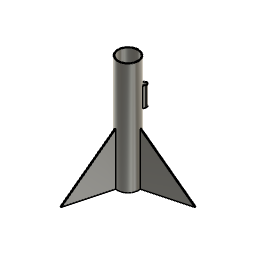
light c11 v1 (Autodesk Fusion 360 design; units mm, degrees)
Autodesk Fusion 360 part; units mm, degrees
sketch "Sketch1" plane through (0, 0, 0) normal (0, 0, 1) x (1, 0, 0)
  circle A0 centre (0, 0) radius 12.5
  circle A1 centre (0, 0) radius 14.5
  line L0 (-110, 110) -> (110, 110)
  line L1 (110, 110) -> (110, -110)
  line L2 (110, -110) -> (-110, -110)
  line L3 (-110, -110) -> (-110, 110)
  line L4 (-110, 110) -> (110, -110) construction
  line L5 (110, 110) -> (-110, -110) construction
  line L6 (-60, 60) -> (-60.3536, 59.6464)
  line L7 (-60.7071, 59.2929) -> (-59.6464, 60.3536)
  line L8 (-58.9393, 60.3536) -> (0.7071, 0.7071)
  line L9 (-60.3536, 58.9393) -> (-0.7071, -0.7071)
  arc A2 (-58.9393, 60.3536) -> (-59.6464, 60.3536) centre (-59.2929, 60) ccw
  arc A3 (-60.3536, 59.6464) -> (-60.3536, 58.9393) centre (-60, 59.2929) ccw
  line L10 (-20.9956, -82.2203) -> (-22.4445, -81.8321)
  arc A4 (-21.4786, -82.0909) -> (-20.8662, -81.7374) centre (-21.3492, -81.608) ccw
  line L11 (-20.8662, -81.7374) -> (0.9659, -0.2588)
  arc A5 (-22.798, -81.2197) -> (-22.4445, -81.8321) centre (-22.3151, -81.3492) ccw
  line L12 (-22.798, -81.2197) -> (-0.9659, 0.2588)
  line L13 (81.7027, 22.9275) -> (82.0909, 21.4786)
  arc A6 (81.8321, 22.4445) -> (81.2197, 22.798) centre (81.3492, 22.3151) ccw
  line L14 (81.2197, 22.798) -> (-0.2588, 0.9659)
  arc A7 (81.7374, 20.8662) -> (82.0909, 21.4786) centre (81.608, 21.3492) ccw
  line L15 (81.7374, 20.8662) -> (0.2588, -0.9659)
  point P0 (-59.2929, 60.7071)
  dimension "d1" = 25
  dimension "d2" = 29
  dimension "d3" = 220
  dimension "d4" = 220
  dimension "d5" = 1
  dimension "d6" = 2
  dimension "d7" = 180
  dimension "d8" = 0.5
  dimension "d10" = 360
  constraint coincident A0.centre A1.centre
  constraint horizontal L0
  constraint perpendicular L0 L1
  constraint parallel L0 L2
  constraint parallel L1 L3
  constraint coincident L4 A0.centre
  constraint coincident L5 A0.centre
  constraint coincident L4 L6.start
  constraint perpendicular L4 L6
  constraint perpendicular L4 L7
  constraint coincident L5 L8.end
  constraint perpendicular L5 L8
  constraint coincident L5 L9.end
  constraint coincident P0 L7
  constraint coincident P0 L8
  constraint tangent L7 A2
  constraint tangent L8 A2
  constraint coincident L7.start L6
  constraint coincident L7.start L9
  constraint tangent L6 A3
  constraint tangent L9 A3
  constraint equal A2 A3
  measures "d1" diameter of A0
  measures "d2" diameter of A1
  measures "d3" distance of L1.end L2.end
  measures "d4" distance of L0.end L1.end
  measures "d5" distance of L6.start L7.start
  measures "d6" distance of L7.start P0
  measures "d7" angle of L8 L9
  measures "d8" radius of A2
extrude "Extrude1" add sketch "Sketch1" along normal blind 70 contours A0 A1 L11 L15 | A0 A1 L14 L15 | A0 A1 L11 L12 | A0 A1 L8 L14 | A0 A1 L9 L12 | A0 A1 L8 L9 makes body 1
sketch "Sketch2" plane through (0, 0, 70) normal (0, 0, 1) x (-1, 0, 0)
  circle A0 centre (0, 0) radius 12.5
  circle A1 centre (0, 0) radius 14.5
  circle A2 centre (0, 0) radius 11
  dimension "d13" = 22
  constraint coincident A0.centre A1.centre
  measures "d13" diameter of A2
extrude "Extrude2" add sketch "Sketch2" along normal blind 2 contours A0 | A1 bodies 1
sketch "Sketch3" plane through (0, 0, 72) normal (0, 0, 1) x (-1, 0, 0)
  circle A0 centre (0, 0) radius 11
  circle A1 centre (0, 0) radius 14.5
  circle A2 centre (0, 0) radius 13.5
  circle A3 centre (0, 0) radius 15
  circle A4 centre (0, 0) radius 16
  dimension "d16" = 27
  dimension "d17" = 30
  dimension "d18" = 32
  constraint coincident A0.centre A1.centre
  constraint concentric A2 A4
  measures "d16" diameter of A2
  measures "d17" diameter of A3
  measures "d18" diameter of A4
extrude "Extrude3" add sketch "Sketch3" along normal blind 100 separate body contours A4 makes body 2
extrude "Extrude4" add sketch "Sketch3" against normal blind 72 contours A3 | A4 bodies 1 2
extrude "Extrude5" add sketch "Sketch1" along normal blind 80 contours A1 L13 A6 L14 A7 L15 | A1 L10 A4 L11 A5 L12 | A1 L6 L7 L8 L9 A2 A3 bodies 1
sketch "Sketch4" plane through (-0.9659, 0.2588, 0) normal (-0.965926, 0.258819, 0) x (-0.258819, -0.965926, 0)
  line L0 (15.9687, 80) -> (15.9687, 0)
  line L1 (15.9687, 0) -> (84.3528, 0)
  line L2 (84.3528, 0) -> (84.3528, 80)
  line L3 (84.3528, 80) -> (15.9687, 80)
  line L4 (15.9687, 80) -> (84.3528, 0)
  line L5 (15.9687, 80) -> (86.3566, 117.9716)
  line L6 (86.3566, 117.9716) -> (140, 40)
  line L7 (140, 40) -> (84.3528, 0)
  constraint coincident L0.start L3.end
  constraint coincident L1.end L2.start
extrude "Extrude6" cut sketch "Sketch4" against normal blind 50 contours L2 L3 L5 L6 L7 | L2 L3 L4 bodies 1
sketch "Sketch5" plane through (-0.7071, -0.7071, 0) normal (-0.707107, -0.707107, 0) x (0.707107, -0.707107, 0)
  line L0 (-15.9687, 0) -> (-15.9687, 80)
  line L1 (-15.9687, 80) -> (-84.3528, 80)
  line L2 (-84.3528, 80) -> (-84.3528, 0)
  line L3 (-84.3528, 0) -> (-15.9687, 0)
  line L4 (-15.9687, 80) -> (-84.3528, 0)
  line L5 (-84.3528, 0) -> (-114.2811, 30.3018)
  line L6 (-114.2811, 30.3018) -> (-99.317, 93.7517)
  line L7 (-99.317, 93.7517) -> (-15.9687, 80)
  constraint coincident L0.end L1.start
  constraint coincident L2.end L3.start
extrude "Extrude7" cut sketch "Sketch5" against normal blind 5 contours L1 L2 L4 | L1 L2 L5 L6 L7 bodies 1
sketch "Sketch6" plane through (-0.2588, 0.9659, 0) normal (-0.258819, 0.965926, 0) x (-0.965926, -0.258819, 0)
  line L0 (-15.9687, 0) -> (-15.9687, 80)
  line L1 (-15.9687, 80) -> (-84.3528, 80)
  line L2 (-84.3528, 80) -> (-84.3528, 0)
  line L3 (-84.3528, 0) -> (-15.9687, 0)
  line L4 (-15.9687, 80) -> (-84.3528, 0)
  line L5 (-135.6724, 47.0573) -> (-84.3528, 0)
  line L6 (-135.6724, 47.0573) -> (-95.0226, 105.2424)
  line L7 (-95.0226, 105.2424) -> (-15.9687, 80)
  constraint coincident L0.end L1.start
  constraint coincident L2.end L3.start
extrude "Extrude8" cut sketch "Sketch6" against normal blind 5 contours L1 L2 L4 | L1 L2 L5 L6 L7 bodies 1
sketch "Sketch7" plane through (0, 0, 0) normal (0, 0, 1) x (1, 0, 0)
  circle A0 centre (8, 17) radius 3
  circle A1 centre (8, 17) radius 4
  line L0 (4.4701, 18.8815) -> (3.3866, 15.4092)
  line L1 (11.85, 15.9148) -> (10, 12)
  line L2 (3.3866, 15.4092) -> (10, 12)
  dimension "d31" = 6
  dimension "d32" = 1
  constraint coincident A1 L0.start
  constraint coincident A1 L1.start
  measures "d31" diameter of A0
extrude "Extrude9" add sketch "Sketch7" along normal blind 100 contours A1 L0 L1 L2 | A1 L0 L2 | A1 L1 L2 bodies 1
sketch "Sketch8" plane through (0, 0, 172) normal (0, 0, 1) x (-1, 0, 0)
  circle A0 centre (0, 0) radius 15
  circle A1 centre (0, 0) radius 16
  circle A2 centre (0, 0) radius 14.5
  dimension "d35" = 29
  constraint coincident A0.centre A1.centre
  measures "d35" diameter of A2
extrude "Extrude10" add sketch "Sketch8" against normal blind 100 contours A0 bodies 1
extrude "Extrude11" cut 1 faces at (10.8115, 14.4974, 100) along direction (0, 0, -1) blind 60 on bodies 1 bodies 1
ref_plane "WorkPlane1" through (8.1388, 17.2026, 100) normal (0, 0, 1) x (1, 0, 0)
sketch "Sketch9" plane through (8.1388, 17.2026, 100) normal (0, 0, 1) x (1, 0, 0)
  arc A0 (2.0285, -4.8484) -> (-0.4161, -3.1897) centre (-8.1388, -17.2026) ccw
  line L0 (2.0285, -4.8484) -> (3.7112, -1.2877)
  arc A1 (3.7112, -1.2877) -> (-3.6687, 1.679) centre (-0.1388, -0.2026) ccw
  line L1 (-3.6687, 1.679) -> (-4.6855, -1.5797)
  arc A2 (-2.2638, -2.3202) -> (-4.6855, -1.5797) centre (-8.1388, -17.2026) ccw
  arc A3 (-0.4161, -3.1897) -> (-2.2638, -2.3202) centre (-0.1388, -0.2026) ccw
extrude "Extrude12" add sketch "Sketch9" along normal blind 30 bodies 1
